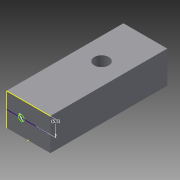
# Autodesk Inventor part: mallet_support
Saved by Autodesk Inventor 2015 (Build 190159000, 159)
## iProperties
Created: 2014-07-15
Part Number: mallet_support
Material: Generic
Document SubType Name: Modeling
Designer: shohei
Density: 1 g/cm^3
Appearance: Default
Mass: 5.73606 g
Surface Area: 25.985 cm^2
Volume: 5.73606 cm^3
Author: shohei
Autodesk Inventor part; units mm, degrees
ref_plane "YZ Plane" through (0, 0, 0) normal (1, 0, 0) x (0, 1, 0)
ref_plane "XZ Plane" through (0, 0, 0) normal (0, 1, 0) x (-1, 0, 0)
ref_plane "XY Plane" through (0, 0, 0) normal (0, 0, 1) x (1, 0, 0)
sketch "Sketch1" plane through (0, 0, 0) normal (0, 0, 1) x (1, 0, 0)
  line L0 (-7.5, 40) -> (7.5, 40)
  line L1 (7.5, 40) -> (7.5, 0)
  line L2 (7.5, 0) -> (-7.5, 0)
  line L3 (-7.5, 0) -> (-7.5, 40)
  line L4 (-10.7602, 0) -> (12.0613, 0) projected
  line L5 (0, -8) -> (0, 48) projected
  point P0 (0, 0)
  dimension "d4" = 7.5
  dimension "d5" = 7.5
  dimension "d6" = 40
  dimension "d7" = 0
  constraints: 8 end point, 2 parallel, 1 horizontal, 1 perpendicular
  measures "d4" distance between parallel lines of L1 L5
  measures "d5" distance between parallel lines of L3 L5
  measures "d6" distance between parallel lines of L0 L4
  measures "d7" distance between parallel lines of L2 L4
extrude "Extrusion1" add sketch "Sketch1" along normal blind 11
sketch "Sketch3" plane through (-7.5, 0, 0) normal (0, -1, 0) x (1, 0, 0)
  line L0 (0, 0) -> (0, 11) projected
  line L1 (0, 5.5) -> (13.8011, 5.5)
  line L2 (0, 11) -> (15, 11) projected
  circle A0 centre (5, 5.5) radius 1
  point P0 (7.5, 0)
  dimension "d11" = 5.5
  dimension "d12" = 2
  constraints: 2 end point, 1 centre point, 1 horizontal, 1 midpoint, 1 point on line
  measures "d11" distance between parallel lines of L2 L1
  measures "d12" diameter of A0
sketch "Sketch4" plane through (0, 0, 11) normal (0, 0, 1) x (1, 0, 0)
  circle A0 centre (0, 30) radius 5
  line L0 (-7.5, 0) -> (7.5, 0) projected
  point P0 (0, 0)
  dimension "d13" = 10
  dimension "d14" = 30
  constraints: 1 centre point
  measures "d13" diameter of A0
  measures "d14" distance from line of L0 A0.centre
extrude "Extrusion3" cut sketch "Sketch4" against normal through all
body "Solid1"
